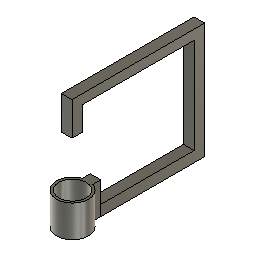
cover encoder (Autodesk Fusion 360 design; units mm, degrees)
Autodesk Fusion 360 part; units mm, degrees
cylinder "CylinderPrimitive1" add diameter 60 height 60 placed x (1, 0, 0) y (0, 1, 0) z (0, 0, 1) at (0, 0, 0) makes body 1
shell "Shell1" thickness 4.5 removed faces 1 at (7.6631, 11.2397, 60) on bodies 1
extrude "Extrude1" cut 1 faces at (5.0863, -5.2303, 4.5) along direction (0, 0, -1) blind 30 on bodies 1 bodies 1
ref_plane "WorkPlane1" through (0, 31, 0) normal (0, 1, 0) x (0, 0, 1)
sketch "Sketch2" plane through (0, 31, 0) normal (0, 1, 0) x (1, 0, 0)
  line L0 (10, 0) -> (-10, 0)
  line L1 (-10, 0) -> (-10, -60)
  line L2 (-10, -60) -> (10, -60)
  line L3 (10, -60) -> (10, 0)
  constraint perpendicular L0 L1
  constraint parallel L0 L2
  constraint parallel L1 L3
  constraint horizontal L0
extrude "Extrude2" add sketch "Sketch2" along normal blind 5 and the other way blind 5 bodies 1
extrude "Extrude3" add 1 faces at (-3.3333, 36, 20) along direction (0, 1, 0) blind 5.3 on bodies 1 bodies 1
extrude "Extrude4" add 1 faces at (-3.3333, 41.3, 20) along direction (0, 1, 0) blind 1.984 on bodies 1 bodies 1
sketch "Sketch3" plane through (0, 0, 0) normal (0, 1, 0) x (1, 0, 0)
ref_plane "WorkPlane2" through (0, 44, 0) normal (0, 1, 0) x (0, 0, 1)
sketch "Sketch4" plane through (0, 44, 0) normal (0, 1, 0) x (1, 0, 0)
  line L0 (10, 0) -> (-10, 0)
  line L1 (-10, 0) -> (-10, -20)
  line L2 (-10, -20) -> (10, -20)
  line L3 (10, -20) -> (10, 0)
  dimension "d17" = 20
  constraint perpendicular L0 L1
  constraint parallel L0 L2
  constraint parallel L1 L3
  constraint horizontal L0
  measures "d17" distance of L0.start L2.end
extrude "Extrude1'" add sketch "Sketch4" along normal blind 55 and the other way blind 1 separate body makes body 2 in component "Component"
extrude "Extrude2'" add 1 faces at (-3.3333, 99, 6.6667) along direction (0, 1, 0) blind 150 on bodies 2 bodies 2 in component "Component"
extrude "Extrude3'" cut 1 faces at (-3.3333, 249, 6.6667) along direction (0, -1, 0) blind 50 on bodies 2 bodies 2 in component "Component"
extrude "Extrude4'" cut 1 faces at (-3.3333, 199, 6.6667) along direction (0, -1, 0) blind 10 on bodies 2 bodies 2 in component "Component"
extrude "Extrude5" add 1 faces at (-3.3333, 189, 6.6667) along direction (0, 1, 0) blind 50 on bodies 2 bodies 2 in component "Component"
sketch "Sketch5" plane through (0, 0, 20) normal (0, 0, 1) x (-1, 0, 0)
  line L0 (10, -239) -> (10, -43)
  line L1 (10, -43) -> (-10, -43)
  line L2 (-10, -43) -> (-10, -239)
  line L3 (-10, -239) -> (10, -239)
  line L4 (10, -239) -> (-10, -239)
  line L5 (-10, -239) -> (-10, -219)
  line L6 (-10, -219) -> (10, -219)
  line L7 (10, -219) -> (10, -239)
  dimension "d30" = 20
  constraint perpendicular L4 L5
  constraint parallel L4 L6
  constraint parallel L5 L7
  constraint coincident L2.end L3.start
  constraint perpendicular L2 L4
  constraint coincident L0.start L3.end
  measures "d30" distance of L0.start L6.end
extrude "Extrude6" add sketch "Sketch5" along normal blind 200 contours L0 L2 L3 L4 L5 L6 L7 bodies 2 in component "Component"
extrude "Extrude7" cut 1 faces at (-3.3333, 232.3333, 220) along direction (0, 0, -1) blind 2 on bodies 2 bodies 2 in component "Component"
sketch "Sketch6" plane through (0, 219, 0) normal (0, -1, 0) x (1, 0, 0)
  line L0 (10, 218) -> (-10, 218)
  line L1 (-10, 218) -> (-10, 20)
  line L2 (-10, 20) -> (10, 20)
  line L3 (10, 20) -> (10, 218)
  line L4 (-10, 218) -> (10, 218)
  line L5 (10, 218) -> (10, 200)
  line L6 (10, 200) -> (-10, 200)
  line L7 (-10, 200) -> (-10, 218)
  constraint horizontal L4
  constraint vertical L5
  constraint horizontal L6
  constraint vertical L7
  constraint coincident L3 L5.end
  constraint coincident L0.end L1.start
extrude "Extrude8" add sketch "Sketch6" along normal blind 220 contours L0 L1 L3 L4 L5 L6 L7 bodies 2 in component "Component"
extrude "Extrude9" add 1 faces at (3.3333, -1, 212) along direction (0, -1, 0) blind 10 on bodies 2 bodies 2 in component "Component"
sketch "Sketch7" plane through (0, 0, 200) normal (0, 0, -1) x (1, 0, 0)
  line L0 (-10, -219) -> (10, -219)
  line L1 (10, -219) -> (10, 11)
  line L2 (10, 11) -> (-10, 11)
  line L3 (-10, 11) -> (-10, -219)
  line L4 (-10, 11) -> (10, 11)
  line L5 (10, 11) -> (10, -9)
  line L6 (10, -9) -> (-10, -9)
  line L7 (-10, -9) -> (-10, 11)
  dimension "d39" = 20
  constraint perpendicular L4 L5
  constraint parallel L4 L6
  constraint parallel L5 L7
  constraint coincident L1.end L2.start
  constraint perpendicular L1 L4
  constraint coincident L2.end L3.start
  measures "d39" distance of L2.end L6.end
extrude "Extrude10" add sketch "Sketch7" along normal blind 45 contours L1 L2 L3 L4 L5 L6 L7 bodies 2 in component "Component"
component "Component" placed x (1, 0, 0) y (0, 1, 0) z (0, 0, 1) at (0, 0, 0)
